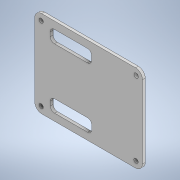
# Autodesk Inventor part: Trippeldekker_Nedre plate
Saved by Autodesk Inventor 2022 (Build 260153000, 153)
## iProperties
Created: 2021-08-25
Part Number: Trippeldekker_Nedre plate
Material: Generic
Document SubType Name: Sheet Metal
Designer: Bruker
Density: 1 g/cm^3
Sheet Metal Rule: Default_mm
Appearance: Default
Author: Bruker
Autodesk Inventor part; units mm, degrees
ref_plane "YZ Plane" through (0, 0, 0) normal (1, 0, 0) x (0, 1, 0)
ref_plane "XZ Plane" through (0, 0, 0) normal (0, 1, 0) x (-1, 0, 0)
ref_plane "XY Plane" through (0, 0, 0) normal (0, 0, 1) x (1, 0, 0)
sketch "Kort" plane through (0, 0, 0) normal (0, 0, 1) x (1, 0, 0)
  line L0 (-3.0921, 63.9853) -> (22.7279, 63.9853)
  line L1 (22.7279, 63.9853) -> (22.7279, 58.9853)
  line L2 (22.7279, 58.9853) -> (-3.0921, 58.9853)
  line L3 (-3.0921, 58.9853) -> (-3.0921, 63.9853)
  line L4 (-2.9921, 20.7153) -> (22.8179, 20.7153)
  line L5 (22.8179, 20.7153) -> (22.8179, 15.7153)
  line L6 (22.8179, 15.7153) -> (-2.9921, 15.7153)
  line L7 (-2.9921, 15.7153) -> (-2.9921, 20.7153)
  line L8 (-14.2921, 69.1953) -> (59.3579, 69.1953)
  line L9 (-14.2921, 10.6153) -> (-14.2921, 69.1953)
  line L10 (59.3579, 10.6153) -> (-14.2921, 10.6153)
  line L11 (59.3579, 69.1953) -> (59.3579, 10.6153)
  circle A0 centre (56.8329, 66.5703) radius 1.575
  circle A1 centre (56.7329, 13.2403) radius 1.575
  circle A2 centre (-11.6671, 66.5703) radius 1.575
  circle A3 centre (-11.6671, 13.2403) radius 1.575
  line L12 (61.3579, 71.1953) -> (-16.2921, 71.1953)
  line L13 (-16.2921, 71.1953) -> (-16.2921, 8.6153)
  line L14 (-16.2921, 8.6153) -> (61.3579, 8.6153)
  line L15 (61.3579, 8.6153) -> (61.3579, 71.1953)
  line L16 (24.7279, 65.9853) -> (-5.0921, 65.9853)
  line L17 (-5.0921, 65.9853) -> (-5.0921, 56.9853)
  line L18 (-5.0921, 56.9853) -> (24.7279, 56.9853)
  line L19 (24.7279, 56.9853) -> (24.7279, 65.9853)
  line L20 (24.8179, 22.7153) -> (-4.9921, 22.7153)
  line L21 (-4.9921, 22.7153) -> (-4.9921, 13.7153)
  line L22 (-4.9921, 13.7153) -> (24.8179, 13.7153)
  line L23 (24.8179, 13.7153) -> (24.8179, 22.7153)
  point P0 (0, 0)
  dimension "d4" = 5.21
  dimension "d5" = 11.2
  dimension "d6" = 5.1
  dimension "d7" = 11.3
  dimension "d8" = 5
  dimension "d9" = 5
  dimension "d10" = 25.82
  dimension "d11" = 25.81
  dimension "d12" = 58.58
  dimension "d13" = 73.65
  dimension "d14" = 2.625
  dimension "d15" = 2.525
  dimension "d16" = 3.15
  dimension "d17" = 3.15
  dimension "d18" = 3.15
  dimension "d19" = 3.15
  dimension "d20" = 2.625
  dimension "d21" = 2.625
  dimension "d22" = 2.625
  dimension "d23" = 2.625
  dimension "d24" = 2.625
  dimension "d25" = 2.625
  dimension "d26" = 2
  dimension "d27" = 2
  dimension "d28" = 2
  constraints: 48 end point, 6 parallel, 4 centre point, 4 perpendicular, 2 horizontal, 1 vertical, 9 other
  measures "d4" distance between parallel lines of L8 L0
  measures "d5" distance between parallel lines of L9 L3
  measures "d6" distance between parallel lines of L10 L6
  measures "d7" distance between parallel lines of L9 L7
  measures "d8" distance between parallel lines of L6 L4
  measures "d9" distance between parallel lines of L0 L2
  measures "d10" distance between parallel lines of L1 L3
  measures "d11" distance between parallel lines of L5 L7
  measures "d12" distance of L8.end L10.start
  measures "d13" distance of L8.start L8.end
  measures "d14" distance from line of L8 A0.centre
  measures "d15" distance from line of L11 A0.centre
  measures "d16" diameter of A0
  measures "d17" diameter of A1
  measures "d18" diameter of A3
  measures "d19" diameter of A2
  measures "d20" distance from line of L8 A2.centre
  measures "d21" distance from line of L9 A2.centre
  measures "d22" distance from line of L10 A3.centre
  measures "d23" distance from line of L9 A3.centre
  measures "d24" distance from line of L10 A1.centre
  measures "d25" distance from line of L11 A1.centre
  measures "d26" distance between parallel lines of L12 L8
  measures "d27" distance between parallel lines of L16 L0
  measures "d28" distance between parallel lines of L20 L4
extrude "Bottom" add sketch "Kort" along normal blind 2 contours L8 L11 L10 L9 | L15 L14 L13 L12
fillet "Kantutjevning" radius 5 4 edges at (61.3579, 8.6153, 1) (61.3579, 71.1953, 1) (-16.2921, 71.1953, 1) (-16.2921, 8.6153, 1)
fillet "Hullkantutjevning" radius 3 8 edges at (-5.0921, 65.9853, 1) (-5.0921, 56.9853, 1) (24.7279, 65.9853, 1) (24.8179, 22.7153, 1) (24.7279, 56.9853, 1) (24.8179, 13.7153, 1) (-4.9921, 13.7153, 1) (-4.9921, 22.7153, 1)
equation "\"BendRadius\" = Thickness"
equation "\"BendReliefWidth\" = Thickness"
equation "\"BendReliefDepth\" = 0.5 * Thickness"
equation "\"CornerReliefSize\" = 4 * Thickness"
equation "\"MinimumRemnant\" = 2 * Thickness"
equation "\"TransitionRadius\" = BendRadius"
equation "\"JacobiRadiusSize\" = BendRadius"
equation "\"GapSize\" = Thickness"
equation "\"Thickness\" = 0.5"
body "Solid1"
